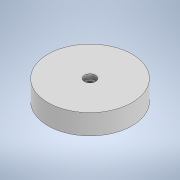
# Autodesk Inventor part: tire_mold_inner
Saved by Autodesk Inventor 2020 (Build 240168000, 168)
## iProperties
Created: 2020-06-07
Part Number: tire_mold_inner
Material: Generic
Document SubType Name: Modeling
Designer: Abhinav Roy
Density: 1 g/cm^3
Appearance: Default
Author: Abhinav Roy
Autodesk Inventor part; units mm, degrees
ref_plane "YZ Plane" through (0, 0, 0) normal (1, 0, 0) x (0, 1, 0)
ref_plane "XZ Plane" through (0, 0, 0) normal (0, 1, 0) x (-1, 0, 0)
ref_plane "XY Plane" through (0, 0, 0) normal (0, 0, 1) x (1, 0, 0)
sketch "Sketch1" plane through (0, 0, 0) normal (0, 1, 0) x (-1, 0, 0)
  circle A0 centre (0, 0) radius 37.5
  dimension "d0" = 75
  constraints: 1 centre point, 1 coincident
  measures "d0" diameter of A0
extrude "Extrusion1" add sketch "Sketch1" along normal blind 18
sketch "Sketch2" plane through (0, 18, 0) normal (0, 1, 0) x (1, 0, 0)
  point P0 (0, 0)
  point P1 (0, 0)
  constraints: 1 coincident
hole "Hole1" at (0, 18, 0) direction (0, -1, 0) diameter 5.2 depth 18 counterbore diameter 10 counterbore depth 4
chamfer "Chamfer1" distance 3 distance2 34 1 edges at (0, 0, -2.6) measured on face at (0, 0.5, -2.6)
body "Solid1"
